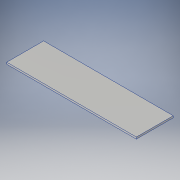
# Autodesk Inventor part: AluminumPlateForWinch
Saved by Autodesk Inventor 2018.2 (Build 222227000, 227)
## iProperties
Created: 2018-01-31
Part Number: AluminumPlateForWinch
Material: Aluminum 6061
Document SubType Name: Modeling
Designer: steele
Mass: 1020.4 g
Surface Area: 1264.92 cm^2
Volume: 377.927 cm^3
Density: 2.7 g/cm^3
Appearance: Aluminum - Flat
Author: steele
Autodesk Inventor part; units mm, degrees
ref_plane "YZ Plane" through (0, 0, 0) normal (1, 0, 0) x (0, 1, 0)
ref_plane "XZ Plane" through (0, 0, 0) normal (0, 1, 0) x (-1, 0, 0)
ref_plane "XY Plane" through (0, 0, 0) normal (0, 0, 1) x (1, 0, 0)
sketch "Sketch1" plane through (0, 0, 0) normal (0, 1, 0) x (-1, 0, 0)
  line L0 (228.6, 65.0875) -> (-228.6, 65.0875)
  line L1 (-228.6, 65.0875) -> (-228.6, -65.0875)
  line L2 (-228.6, -65.0875) -> (228.6, -65.0875)
  line L3 (228.6, -65.0875) -> (228.6, 65.0875)
  line L4 (228.6, 65.0875) -> (-228.6, -65.0875) construction
  line L5 (-228.6, 65.0875) -> (228.6, -65.0875) construction
  point P0 (0, 0)
  dimension "d0" = 457.2
  dimension "d1" = 130.175
  constraints: 12 end point, 2 midpoint, 2 parallel, 1 horizontal, 1 perpendicular
  measures "d0" distance of L0.start L0.end
  measures "d1" distance of L1.end L0.end
extrude "Extrusion1" add sketch "Sketch1" along normal blind 6.35
body "Solid1"
